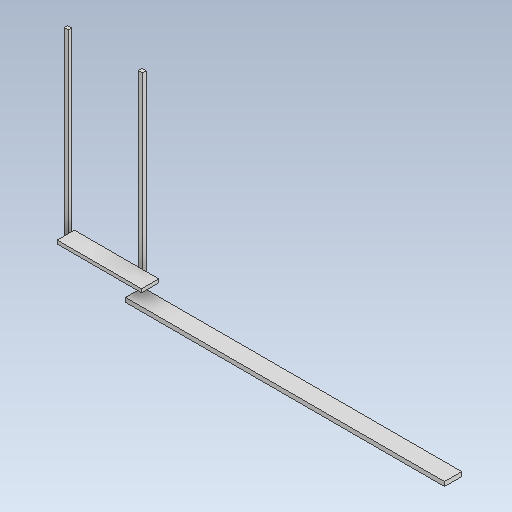
# Autodesk Inventor part: side_bumper
Saved by Autodesk Inventor 2020 (Build 240168000, 168)
## iProperties
Created: 2022-07-15
Part Number: side_bumper
Material: 일반
Document SubType Name: Modeling
Designer: SeungJin
Density: 1 g/cm^3
Appearance: 기본값
Author: SeungJin
Autodesk Inventor part; units mm, degrees
ref_plane "YZ Plane" through (0, 0, 0) normal (1, 0, 0) x (0, 1, 0)
ref_plane "XZ Plane" through (0, 0, 0) normal (0, 1, 0) x (-1, 0, 0)
ref_plane "XY Plane" through (0, 0, 0) normal (0, 0, 1) x (1, 0, 0)
sketch "스케치1" plane through (0, 0, 0) normal (0, 0, 1) x (1, 0, 0)
  line L0 (-40.635, -22.4556) -> (-28.635, -22.4556) projected
  line L1 (-40.635, -22.4556) -> (-40.635, 517.5444) projected
  line L2 (-28.635, 517.5444) -> (-40.635, 517.5444) projected
  line L3 (-28.635, -22.4556) -> (-28.635, 517.5444) projected
  line L4 (-58.635, -22.4556) -> (0, -22.4556) projected
  line L5 (-58.635, -22.4556) -> (-58.635, 517.5444) projected
  line L6 (-46.635, 517.5444) -> (-58.635, 517.5444) projected
  line L7 (-46.635, 0) -> (-46.635, 517.5444) projected
  line L8 (18, 22.5444) -> (18, 12.5098) projected
  line L9 (18, 12.5098) -> (18, -270) projected
  line L10 (-239.1749, -22.4556) -> (-227.1749, -22.4556) projected
  line L11 (-239.1749, -22.4556) -> (-239.1749, 517.5444) projected
  line L12 (-227.1749, 517.5444) -> (-239.1749, 517.5444) projected
  line L13 (-227.1749, -22.4556) -> (-227.1749, 517.5444) projected
  line L14 (-257.1749, -22.4556) -> (-245.1749, -22.4556) projected
  line L15 (-257.1749, -22.4556) -> (-257.1749, 517.5444) projected
  line L16 (-245.1749, 517.5444) -> (-257.1749, 517.5444) projected
  line L17 (-245.1749, -22.4556) -> (-245.1749, 517.5444) projected
  line L18 (18, 22.5444) -> (-257.1749, 22.5444)
  line L19 (-257.1749, 22.5444) -> (-257.1749, -37.4556)
  line L20 (-257.1749, -37.4556) -> (18, -37.4556)
  line L21 (18, -37.4556) -> (18, 22.5444)
  line L22 (18, 12.5444) -> (-257.1749, 12.5444)
  point P0 (0, 0)
  dimension "d0" = 60
  dimension "d1" = 10
  constraints: 10 end point, 3 point on line, 2 parallel, 2 perpendicular, 1 horizontal, 2 other
  measures "d0" distance of L19.end L18.end
  measures "d1" distance between parallel lines of L22 L18
extrude "돌출1" add sketch "스케치1" along normal blind 10 and the other way blind 50 contours L22 L7 L18 L1 | L1 L18 L3 L22 | L3 L18 L8 L22 | L22 L5 L18 L7 | L22 L13 L18 L5 | L22 L11 L18 L13 | L22 L17 L18 L11 | L22 L15 L18 L17
sketch "스케치2" plane through (-257.1749, 22.5444, 10) normal (0, 1, 0) x (1, 0, 0)
  line L0 (0, 60) -> (0, 0) projected
  line L1 (275.1749, 0) -> (0, 0) projected
  line L2 (275.1749, 60) -> (275.1749, 0) projected
  line L3 (0, 60) -> (275.1749, 60) projected
  circle A0 centre (-63.5, -41.3) radius 75.8469 projected
  line L4 (-155.5399, 160) -> (-155.5399, 53) projected
  line L5 (-139.3469, -41.3) -> (-155.5399, -41.3)
  line L6 (0, 0) -> (275.1749, 0) projected
  line L7 (30, 0) -> (30, 60)
  line L8 (0, 60) -> (0, 0) projected
  line L9 (30, 0) -> (0, 0)
  line L10 (0, 0) -> (0, -40)
  line L11 (0, -40) -> (30, -40)
  line L12 (30, -40) -> (30, 0)
  point P0 (257.1749, 10)
  point P1 (0, 40)
  point P2 (30, 40)
  dimension "d7" = 16.193
  dimension "d8" = 40
  dimension "d44" = 30
  constraints: 12 end point, 4 point on line, 3 perpendicular, 2 parallel, 1 horizontal, 1 horizontal alignment, 1 other
  measures "d7" distance of L5.start L5.end
  measures "d8" distance of L9.end L10.end
  measures "d44" distance between parallel lines of L7 L0
extrude "돌출2" cut sketch "스케치2" against normal through all contours L3 L7 L1 A0 L0 | A0 L1 L0 | L1 A0 L11 L10 | L1 L12 L11 A0
ref_plane "작업 평면1" through (1096.6045, -22.4556, -50) normal (0, 0, -1) x (-1, 0, 0)
sketch "스케치3" plane through (1096.6045, -22.4556, -50) normal (0, 0, -1) x (-1, 0, 0)
  line L0 (1323.7794, 35) -> (1078.6045, 35) projected
  line L1 (1078.6045, 35) -> (1078.6045, 45) projected
  line L2 (1078.6045, 45) -> (1323.7794, 45) projected
  line L3 (1353.7794, 35) -> (1078.6045, 35) projected
  line L4 (1353.7794, 0) -> (1341.7794, 0) projected
  line L5 (1353.7794, 0) -> (1353.7794, 540) projected
  line L6 (1341.7794, 540) -> (1353.7794, 540) projected
  line L7 (1341.7794, 0) -> (1341.7794, 540) projected
  line L8 (1335.7794, 0) -> (1323.7794, 0) projected
  line L9 (1335.7794, 0) -> (1335.7794, 540) projected
  line L10 (1323.7794, 540) -> (1335.7794, 540) projected
  line L11 (1323.7794, 0) -> (1323.7794, 540) projected
  line L12 (1155.2395, 0) -> (1096.6045, 0) projected
  line L13 (1155.2395, 0) -> (1155.2395, 540) projected
  line L14 (1143.2395, 540) -> (1155.2395, 540) projected
  line L15 (1143.2395, 22.4556) -> (1143.2395, 540) projected
  line L16 (1137.2395, 0) -> (1125.2395, 0) projected
  line L17 (1137.2395, 0) -> (1137.2395, 540) projected
  line L18 (1125.2395, 540) -> (1137.2395, 540) projected
  line L19 (1125.2395, 0) -> (1125.2395, 540) projected
  line L20 (1078.6045, 35) -> (1353.7794, 35)
  line L21 (1353.7794, 35) -> (1353.7794, -15)
  line L22 (1353.7794, -15) -> (1078.6045, -15)
  line L23 (1078.6045, -15) -> (1078.6045, 35)
  line L24 (1323.7794, 45) -> (1323.7794, 35) projected
  point P0 (1096.6045, 22.4556)
  point P1 (198.5399, -62.5444)
  point P2 (198.5399, -12.5444)
  point P3 (1353.7794, -12.5444)
  point P4 (186.5399, -62.5444)
  point P5 (1137.2395, 35)
  point P6 (1125.2395, 35)
  point P7 (198.5399, 0)
  point P8 (186.5399, 0)
  point P9 (198.5399, 0)
  point P10 (186.5399, 0)
  dimension "d11" = 50
  constraints: 8 end point, 2 parallel, 1 horizontal, 1 perpendicular, 1 point on line, 1 other
  measures "d11" distance of L21.end L20.end
extrude "돌출3" add sketch "스케치3" along normal blind 10 contours L7 L6 L5 L3 | L3 L5 L4 L7 | L17 L12 L19 L0 | L0 L19 L2 L17 | L2 L19 L18 L17
ref_plane "작업 평면2" through (-12, -260, -30) normal (0, 0, -1) x (0, 1, 0)
sketch "스케치4" plane through (1096.6045, -22.4556, -50) normal (0, 0, 1) x (1, 0, 0)
  line L0 (-1143.2395, 260) -> (-1155.2395, 260)
  line L1 (-1155.2395, 0) -> (-1155.2395, 260)
  line L2 (-1096.6045, 0) -> (-1155.2395, 0)
  line L3 (-1143.2395, 22.4556) -> (-1143.2395, 260)
  line L4 (-1125.2395, 260) -> (-1137.2395, 260)
  line L5 (-1137.2395, 0) -> (-1137.2395, 260)
  line L6 (-1125.2395, 0) -> (-1137.2395, 0)
  line L7 (-1125.2395, 0) -> (-1125.2395, 260)
  line L8 (-1125.2395, 45) -> (-1078.6045, 45)
  line L9 (-1078.6045, 45) -> (-1078.6045, 35)
  line L10 (-1137.2395, 35) -> (-1323.7794, 35)
  line L11 (-198.5399, -12.5444) -> (-168.5399, -12.5444)
  line L12 (-198.5399, -22.5444) -> (-198.5399, -12.5444)
  line L13 (-168.5399, -22.5444) -> (-198.5399, -22.5444)
  line L14 (-168.5399, -22.5444) -> (-168.5399, -12.5444)
  line L15 (-1341.7794, 260) -> (-1353.7794, 260)
  line L16 (-1353.7794, 0) -> (-1353.7794, 260)
  line L17 (-1341.7794, 0) -> (-1353.7794, 0)
  line L18 (-1341.7794, 0) -> (-1341.7794, 260)
  line L19 (-1323.7794, 260) -> (-1335.7794, 260)
  line L20 (-1335.7794, 0) -> (-1335.7794, 260)
  line L21 (-1323.7794, 0) -> (-1335.7794, 0)
  line L22 (-1323.7794, 0) -> (-1323.7794, 260)
  line L23 (-1125.2395, 0) -> (-198.5399, 0)
  line L24 (-198.5399, 0) -> (-198.5399, -12.5444)
  line L25 (-198.5399, -12.5444) -> (-1125.2395, -12.5444)
  line L26 (-1125.2395, -12.5444) -> (-1125.2395, 0)
  line L27 (-1353.7794, 0) -> (-1353.7794, 540)
  line L28 (-1125.2395, 540) -> (-1125.2395, 45)
  line L29 (-1125.2395, 0) -> (-896.6996, 0)
  line L30 (-896.6996, 0) -> (-896.6996, -62.5444)
  line L31 (-896.6996, -62.5444) -> (-1125.2395, -62.5444)
  line L32 (-1125.2395, -62.5444) -> (-1125.2395, 0)
  line L33 (-896.6996, -62.5444) -> (-198.5399, -62.5444)
  line L34 (-99.27, -25.0888) -> (-69.27, -25.0888)
  line L35 (-69.27, -25.0888) -> (-69.27, -62.5444)
  line L36 (-69.27, -62.5444) -> (-99.27, -62.5444)
  line L37 (-99.27, -62.5444) -> (-99.27, -25.0888)
  line L38 (-99.27, -25.0888) -> (-69.27, -62.5444) construction
  line L39 (-69.27, -25.0888) -> (-99.27, -62.5444) construction
  line L40 (-1323.7794, 0) -> (-1323.7794, -12.5444)
  line L41 (-1353.7794, 540) -> (-1341.7794, 540)
  line L42 (-1341.7794, 0) -> (-1353.7794, 0)
  line L43 (-1341.7794, 540) -> (-1341.7794, 0)
  line L44 (-1137.2395, 0) -> (-1137.2395, 35)
  line L45 (-1125.2395, 0) -> (-1137.2395, 0)
  line L46 (-1137.2395, 540) -> (-1125.2395, 540)
  line L47 (-1125.2395, 35) -> (-1137.2395, 35)
  line L48 (-1125.2395, 35) -> (-1125.2395, 0)
  line L49 (-1137.2395, 45) -> (-1125.2395, 45)
  line L50 (-1137.2395, 45) -> (-1137.2395, 540)
  line L51 (-1125.2395, 35) -> (-1125.2395, 45)
  line L52 (-1078.6045, 35) -> (-1125.2395, 35)
  line L53 (-1137.2395, 45) -> (-1137.2395, 35)
  line L54 (-1323.7794, 45) -> (-1137.2395, 45)
  line L55 (-1323.7794, 35) -> (-1323.7794, 45)
  point P0 (-1096.6045, 22.4556)
  point P1 (-1125.2395, -12.5444)
  point P2 (-174.5399, 0)
  point P3 (-1028.9695, 0)
  point P4 (-962.6996, 0)
  point P5 (-168.5399, 0)
  point P6 (-180.5399, 0)
  point P7 (-186.5399, 0)
  point P8 (-84.27, -43.8166)
  point P9 (-69.27, 0)
  point P10 (-168.5399, 0)
  point P11 (-99.27, 0)
  point P12 (-962.6996, 0)
  point P13 (-168.5399, 0)
  point P14 (-1323.7794, -12.5444)
  point P15 (-84.27, 0)
  point P16 (-294.8099, -22.5444)
  point P17 (-294.8099, -12.5444)
extrude "돌출4" add sketch "스케치4" along normal blind 50 contours L2 L23 L30 L25 L26 | L23 L24 L25 L30
ref_plane "작업 평면3" through (-210.5399, 20.5444, 10) normal (0, 1, 0) x (1, 0, 0)
sketch "스케치7" plane through (1096.6045, -22.4556, -50) normal (0, 0, 1) x (1, 0, 0)
  line L0 (0, -260) -> (12, -260) projected
  line L1 (12, 0) -> (12, -260) projected
  line L2 (0, 0) -> (12, 0) projected
  line L3 (0, 0) -> (0, -260) projected
  line L4 (18, -260) -> (30, -260) projected
  line L5 (30, 0) -> (30, -260) projected
  line L6 (18, 0) -> (30, 0) projected
  line L7 (18, 0) -> (18, -260) projected
  line L8 (-1307.1444, -12.5444) -> (-1323.7794, -12.5444) projected
  line L9 (-198.5399, -22.5444) -> (-198.5399, 35) projected
  line L10 (-168.5399, -22.5444) -> (-198.5399, -22.5444) projected
  line L11 (-168.5399, -22.5444) -> (-168.5399, 35) projected
  line L12 (-1078.6045, -12.5444) -> (-1307.1444, -12.5444) projected
  line L13 (0, 12.5444) -> (30, 12.5444)
  line L14 (30, 12.5444) -> (30, 0)
  line L15 (30, 0) -> (0, 0)
  line L16 (0, 0) -> (0, 12.5444)
  point P0 (-1096.6045, 22.4556)
  point P1 (-1323.7794, 35)
  point P2 (-1307.1444, 35)
  point P3 (-198.5399, 12.5444)
  point P4 (30, 12.5444)
  point P5 (0, 12.5444)
  point P6 (-198.5399, -12.5444)
  point P7 (-1078.6045, 35)
  constraints: 8 end point, 2 parallel, 1 horizontal, 1 perpendicular, 2 other
extrude "돌출7" [suppressed]
sketch "스케치12" plane through (0, 0, 10) normal (0, 0, 1) x (1, 0, 0)
  line L0 (-180.5399, 0) -> (-12, 0)
  line L1 (-227.1749, 22.5444) -> (-40.635, 22.5444) projected
  line L2 (18, 22.5444) -> (18, 12.5444) projected
  line L3 (898.0646, -22.4556) -> (-28.635, -22.4556) projected
  line L4 (898.0646, -35) -> (898.0646, -22.4556) projected
  line L5 (-40.635, 12.5444) -> (-227.1749, 12.5444) projected
  line L6 (-28.635, -22.4556) -> (-28.635, -35) projected
  line L7 (-28.635, -35) -> (898.0646, -35) projected
  line L8 (-28.635, 12.5444) -> (-28.635, 22.5444) projected
  line L9 (-28.635, 22.5444) -> (18, 22.5444) projected
  line L10 (18, 12.5444) -> (-28.635, 12.5444) projected
  line L11 (-40.635, 22.5444) -> (-40.635, 12.5444) projected
  line L12 (-227.1749, 12.5444) -> (-227.1749, 22.5444) projected
  point P0 (0, 0)
  point P1 (-145.9049, -22.4556)
  point P2 (-46.635, -22.4556)
  point P3 (114.27, 0)
  point P4 (-114.27, 0)
  point P5 (18, 12.5444)
  point P6 (114.27, 12.5444)
  point P7 (114.27, 0)
  point P8 (114.27, 0)
  point P9 (114.27, 12.5444)
  point P10 (114.27, 12.5444)
  point P11 (114.27, 12.5444)
  point P12 (114.27, 12.5444)
  point P13 (114.27, 12.5444)
  point P14 (114.27, 12.5444)
  point P15 (114.27, 12.5444)
  point P16 (114.27, 12.5444)
  point P17 (114.27, 12.5444)
  point P18 (-28.635, -35)
  constraints: 2 end point, 1 horizontal
hole "구멍1" [suppressed]
sketch "스케치13" plane through (0, 0, 10) normal (0, 0, 1) x (1, 0, 0)
  line L0 (-81.27, 0) -> (-81.27, -37.4556) projected
  line L1 (-111.27, -37.4556) -> (-111.27, 0) projected
  line L2 (-180.5399, 0) -> (-180.5399, -37.4556) projected
  line L3 (-12, -37.4556) -> (-12, 0) projected
  line L4 (-111.27, 0) -> (-81.27, 0) projected
  line L5 (-12, 0) -> (18, 0) projected
  line L6 (-210.5399, 0) -> (-180.5399, 0) projected
  point P0 (0, 0)
  point P1 (-195.5399, -18.7278)
  point P2 (-96.27, -18.7278)
  point P3 (3, -18.7278)
hole "구멍2" [suppressed]
sketch "스케치14" plane through (0, 0, -50) normal (0, 0, -1) x (-1, 0, 0)
  line L0 (227.1749, 22.5444) -> (40.635, 22.5444) projected
  line L1 (-18, 22.5444) -> (-18, 12.5444) projected
  line L2 (210.5399, 62.5444) -> (-18, 62.5444) projected
  line L3 (-18, 0) -> (180.5399, 0) projected
  line L4 (12, -37.4556) -> (-18, -37.4556)
  line L5 (-18, -37.4556) -> (-18, 0)
  line L6 (-18, 0) -> (12, 0)
  line L7 (12, 0) -> (12, -37.4556)
  line L8 (81.27, -37.4556) -> (81.27, 0) projected
  line L9 (111.27, -37.4556) -> (81.27, -37.4556)
  line L10 (81.27, -37.4556) -> (81.27, 0)
  line L11 (81.27, 0) -> (111.27, 0)
  line L12 (111.27, 0) -> (111.27, -37.4556)
  line L13 (210.5399, 62.5444) -> (-18, 62.5444) projected
  line L14 (227.1749, 12.5444) -> (227.1749, 22.5444) projected
  line L15 (210.5399, 62.5444) -> (180.5399, 62.5444)
  line L16 (180.5399, 62.5444) -> (180.5399, 0)
  line L17 (180.5399, 0) -> (210.5399, 0)
  line L18 (210.5399, 0) -> (210.5399, 62.5444)
  line L19 (40.635, 12.5444) -> (227.1749, 12.5444) projected
  line L20 (28.635, 12.5444) -> (28.635, 22.5444) projected
  line L21 (28.635, 22.5444) -> (-18, 22.5444) projected
  line L22 (-18, 12.5444) -> (28.635, 12.5444) projected
  line L23 (40.635, 22.5444) -> (40.635, 12.5444) projected
  line L24 (227.1749, 12.5444) -> (227.1749, 22.5444) projected
  point P0 (0, 0)
  point P1 (180.5399, -37.4556)
  point P2 (-18, 62.5444)
  point P3 (-18, -37.4556)
  point P4 (191.7766, 0)
  point P5 (180.5399, -37.4556)
  point P6 (180.5399, 22.5444)
  point P7 (180.5399, 12.5444)
  constraints: 24 end point, 6 parallel, 3 horizontal, 3 perpendicular, 1 point on line, 4 other
extrude "돌출10" [suppressed]
sketch "스케치15" plane through (0, 0, -50) normal (0, 0, -1) x (-1, 0, 0)
  circle A0 centre (96.27, -18.7278) radius 2.25 projected
  circle A1 centre (195.5399, -18.7278) radius 2.25 projected
  circle A2 centre (-3, -18.7278) radius 2.25 projected
  circle A3 centre (-3, -18.7278) radius 2.25 projected
  point P0 (0, 0)
  constraints: 3 coincident
hole "구멍3" [suppressed]
sketch "스케치16" plane through (0, 0, 10) normal (0, 0, 1) x (1, 0, 0)
  line L0 (18, 12.5444) -> (18, 22.5444) projected
  line L1 (18, 22.5444) -> (-227.1749, 22.5444) projected
  line L2 (-227.1749, 12.5444) -> (18, 12.5444) projected
  line L3 (-227.1749, 22.5444) -> (-227.1749, 12.5444) projected
  point P0 (0, 0)
extrude "돌출11" cut sketch "스케치16" against normal blind 10
sketch "스케치17" plane through (-180.5399, 22.5444, -30) normal (0, 0, -1) x (-1, 0, 0)
  line L0 (30, 0) -> (30, -10) projected
  line L1 (0, 0) -> (30, 0) projected
  line L2 (0, 0) -> (0, -10) projected
  line L3 (30, -10) -> (0, -10) projected
  point P0 (-180.5399, -22.5444)
extrude "돌출12" [suppressed]
